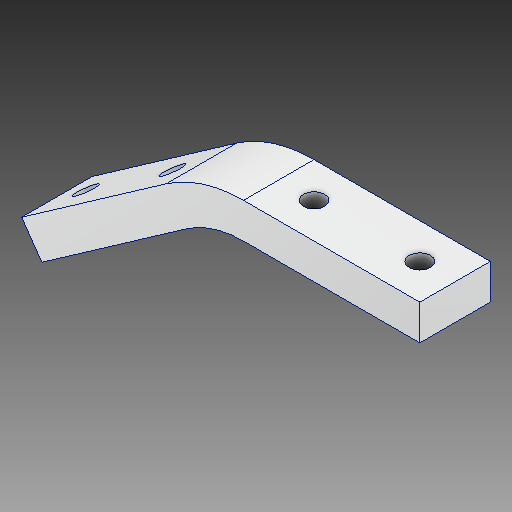
# Autodesk Inventor part: カウンター1.2.1
Saved by Autodesk Inventor 2020 (Build 240168000, 168)
## iProperties
Created: 2019-09-03
Part Number: カウンター1.2.1
Material: アルミニウム 6061
Document SubType Name: Modeling
Designer: 雪村
Density: 2.7 g/cm^3
Appearance: アルミニウム - フラット
Mass: 7.73952 g
Surface Area: 20.3666 cm^2
Volume: 2.86649 cm^3
Author: 雪村
Autodesk Inventor part; units mm, degrees
ref_plane "YZ Plane" through (0, 0, 0) normal (1, 0, 0) x (0, 1, 0)
ref_plane "XZ Plane" through (0, 0, 0) normal (0, 1, 0) x (-1, 0, 0)
ref_plane "XY Plane" through (0, 0, 0) normal (0, 0, 1) x (1, 0, 0)
sketch "スケッチ1" plane through (0, 0, 0) normal (0, 0, 1) x (1, 0, 0)
  line L0 (0, 0) -> (25, 0)
  line L1 (25, 0) -> (25, 5)
  line L2 (25, 5) -> (0, 5)
  line L3 (0, 5) -> (0, 0)
  circle A0 centre (5, 2.5) radius 1.5 construction
  circle A1 centre (20, 2.5) radius 1.5 construction
  line L4 (20, 2.5) -> (5, 2.5) construction
  line L5 (-10.9711, 1.5408) -> (-31.4499, -12.7986)
  line L6 (-31.4499, -12.7986) -> (-28.582, -16.8943)
  line L7 (-28.582, -16.8943) -> (-8.1032, -2.5549)
  line L8 (-8.1032, -2.5549) -> (-10.9711, 1.5408)
  line L9 (-30.016, -14.8465) -> (-9.5372, -0.5071) construction
  arc A2 (0, 2.5) -> (-9.5372, -0.5071) centre (0, -14.1275) ccw construction
  arc A3 (0, 5) -> (-10.9711, 1.5408) centre (0, -14.1275) ccw
  arc A4 (0, 0) -> (-8.1032, -2.5549) centre (0, -14.1275) ccw
  circle A5 centre (-25.9202, -11.9786) radius 1.5 construction
  circle A6 centre (-13.6329, -3.3749) radius 1.5 construction
  point P0 (25, 2.5)
  point P1 (-8.1032, -2.5549)
  point P2 (-10.9711, 1.5408)
  dimension "d0" = 5
  dimension "d1" = 3
  dimension "d2" = 3
  dimension "d3" = 15
  dimension "d4" = 5
  dimension "d5" = 5
  dimension "d6" = 5
  dimension "d7" = 25
  dimension "d8" = 2.5
  dimension "d9" = 2.5
  dimension "d10" = 145
  dimension "d11" = 10
  dimension "d12" = 3
  dimension "d13" = 3
  dimension "d14" = 5
  dimension "d15" = 5
  constraints: 20 end point, 7 centre point, 6 point on circle, 4 midpoint, 4 point on line, 2 horizontal, 2 horizontal alignment, 2 parallel, 2 tangent, 2 vertical, 1 perpendicular
  measures "d0" distance of L1.end L0.end
  measures "d1" diameter of A0
  measures "d2" diameter of A1
  measures "d3" distance of L4.start L4.end
  measures "d4" distance from line of L3 L4.end
  measures "d5" distance from line of L1 L4.start
  measures "d6" distance of L6.end L5.end
  measures "d7" distance of L5.start L5.end
  measures "d8" radial gap between concentric circles of A2 A3
  measures "d9" radial gap between concentric circles of A2 A4
  measures "d10" angle of L4 L9
  measures "d11" distance of L9.end A2.start
  measures "d12" diameter of A5
  measures "d13" diameter of A6
  measures "d14" distance from line of A6.centre L8
  measures "d15" distance from line of L6 A5.centre
extrude "押し出し1" add sketch "スケッチ1" along normal blind 10
sketch "スケッチ2" plane through (0, 0, 0) normal (0, -1, 0) x (1, 0, 0)
  line L0 (25, 0) -> (25, 10) projected
  circle A0 centre (5, 5) radius 1.5
  circle A1 centre (20, 5) radius 1.5
  point P0 (0, 0)
  point P1 (25, 5)
  dimension "d18" = 3
  dimension "d19" = 3
  dimension "d20" = 15
  dimension "d21" = 5
  constraints: 2 centre point, 2 horizontal alignment, 1 midpoint
  measures "d18" diameter of A0
  measures "d19" diameter of A1
  measures "d20" distance of A1.centre A0.centre
  measures "d21" distance from line of L0 A1.centre
extrude "押し出し2" cut sketch "スケッチ2" against normal through all
sketch "スケッチ3" plane through (-8.1032, -2.5549, 0) normal (0.5736, -0.8192, 0) x (0.8192, 0.5736, 0)
  line L0 (-25, 0) -> (-25, 10) projected
  circle A0 centre (-20, 5) radius 1.5
  circle A1 centre (-5, 5) radius 1.5
  point P0 (8.1032, 0)
  point P1 (-25, 5)
  dimension "d24" = 3
  dimension "d25" = 3
  dimension "d26" = 15
  dimension "d27" = 5
  constraints: 2 centre point, 2 horizontal alignment, 1 midpoint
  measures "d24" diameter of A0
  measures "d25" diameter of A1
  measures "d26" distance of A1.centre A0.centre
  measures "d27" distance from line of L0 A0.centre
extrude "押し出し3" cut sketch "スケッチ3" against normal through all
